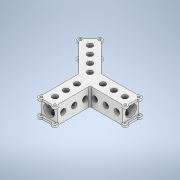
# Autodesk Inventor part: BracketV2
Saved by Autodesk Inventor 2022 (Build 260153000, 153)
## iProperties
Created: 2022-02-05
Part Number: BracketV2
Material: Generic
Document SubType Name: Modeling
Designer: ultra
Density: 1 g/cm^3
Appearance: Smooth - White
Author: ultra
Autodesk Inventor part; units mm, degrees
ref_plane "YZ Plane" through (0, 0, 0) normal (1, 0, 0) x (0, 1, 0)
ref_plane "XZ Plane" through (0, 0, 0) normal (0, 1, 0) x (-1, 0, 0)
ref_plane "XY Plane" through (0, 0, 0) normal (0, 0, 1) x (1, 0, 0)
sketch "Sketch2" plane through (0, 0, 0) normal (1, 0, 0) x (0, 1, 0)
  circle A0 centre (0, 0) radius 12.881
  line L0 (-16, -18.5) -> (16, -18.5)
  line L1 (16, -18.5) -> (16, 18.5)
  line L2 (16, 18.5) -> (-16, 18.5)
  line L3 (-16, 18.5) -> (-16, -18.5)
  line L4 (-16, -18.5) -> (16, 18.5) construction
  line L5 (16, -18.5) -> (-16, 18.5) construction
  dimension "d9" = 25.762
  dimension "d10" = 32
  dimension "d11" = 37
  constraints: 12 end point, 2 midpoint, 2 parallel, 1 centre point, 1 coincident, 1 horizontal, 1 perpendicular
  measures "d9" diameter of A0
  measures "d10" distance of L2.end L1.end
  measures "d11" distance of L1.end L0.end
extrude "Extrusion2" add sketch "Sketch2" along normal blind 76.2
sketch "Sketch3" plane through (0, -16, -18.5) normal (0, 0, -1) x (-1, 0, 0)
  line L0 (0, 0) -> (0, 32) projected
  circle A0 centre (18.5, 16) radius 12.881
  line L1 (0, 32) -> (0, 0)
  line L2 (0, 0) -> (37, 0)
  line L3 (37, 0) -> (37, 32)
  line L4 (37, 32) -> (0, 32)
  line L5 (0, 32) -> (37, 0) construction
  line L6 (0, 0) -> (37, 32) construction
  point P0 (0, 16)
  dimension "d14" = 25.762
  dimension "d15" = 32
  dimension "d16" = 37
  constraints: 12 end point, 2 midpoint, 2 parallel, 1 centre point, 1 coincident, 1 perpendicular
  measures "d14" diameter of A0
  measures "d15" distance of L3.end L2.end
  measures "d16" distance of L2.end L1.end
extrude "Extrusion3" add sketch "Sketch3" against normal blind 113.2
sketch "Sketch4" plane through (76.2, -16, -18.5) normal (0, 0, -1) x (-1, 0, 0)
  circle A0 centre (94.7, 16) radius 12.881 projected
  point P0 (76.2, 16)
extrude "Extrusion4" add sketch "Sketch4" against normal blind 37
sketch "Sketch5" plane through (76.2, 16, 18.5) normal (0, 1, 0) x (1, 0, 0)
  line L0 (-113.2, 37) -> (0, 37) projected
  line L1 (-113.2, 37) -> (-113.2, -76.2) projected
  line L2 (-113.2, 37) -> (-100.1185, 50.0815)
  line L3 (-113.2, 37) -> (-94.7, 37) construction
  line L4 (-113.2, 37) -> (-126.2815, 23.9185)
  line L5 (-113.2, 37) -> (-94.7, 37) construction
  line L6 (-100.1185, 50.0815) -> (-154.0001, 103.963)
  line L7 (-126.2815, 23.9185) -> (-180.163, 77.8001)
  line L8 (-126.2815, 23.9185) -> (-50.0815, 23.9185) construction
  line L9 (-154.0001, 103.963) -> (-180.163, 77.8001)
  line L10 (-100.1185, 50.0815) -> (-87.037, 37)
  line L11 (-126.2815, 23.9185) -> (-113.2, 10.837)
  point P0 (-76.2, 18.5)
  dimension "d21" = 18.5
  dimension "d22" = 45
  dimension "d23" = 18.5
  dimension "d24" = 135
  dimension "d25" = 76.2
  dimension "d26" = 76.2
  dimension "d27" = 135
  constraints: 20 end point, 3 equal length, 3 horizontal, 2 point on line
  measures "d21" distance of L0.start L2.end
  measures "d22" angle of L3 L2
  measures "d23" distance of L0.start L4.end
  measures "d24" angle of L4 L5
  measures "d25" distance of L2.end L6.end
  measures "d26" distance of L4.end L7.end
  measures "d27" angle of L8 L7
extrude "Extrusion5" add sketch "Sketch5" against normal blind 32
sketch "Sketch7" plane through (-77.8001, -16, -85.463) normal (-0.7071068, 0, -0.7071068) x (-0.7071068, 0, 0.7071068)
  line L0 (36.4256, 0.4968) -> (36.4256, 31.5032)
  line L1 (36.4256, 31.5032) -> (0.5744, 31.5032)
  line L2 (0.5744, 31.5032) -> (0.5744, 0.4968)
  line L3 (0.5744, 0.4968) -> (36.4256, 0.4968)
  circle A0 centre (18.5, 16) radius 12.881
  point P0 (5.4185, 16)
  point P1 (36.4256, 16)
  dimension "d131" = 25.762
  constraints: 8 end point, 1 centre point
  measures "d131" diameter of A0
extrude "Extrusion6" cut sketch "Sketch7" against normal blind 101.6 contours A0
sketch "Sketch8" plane through (76.2, 16, 18.5) normal (0, 1, 0) x (1, 0, 0)
  line L0 (-76.2, 0) -> (0, 0) projected
  line L1 (-87.037, 37) -> (0, 37) projected
  line L2 (-87.037, 37) -> (-154.0001, 103.963) projected
  line L3 (-180.163, 77.8001) -> (-113.2, 10.837) projected
  line L4 (-113.2, 10.837) -> (-113.2, -76.2) projected
  line L5 (-76.2, 0) -> (-76.2, -76.2) projected
  line L6 (0, 37) -> (5, 37)
  line L7 (5, 37) -> (5, 0)
  line L8 (5, 0) -> (0, 0)
  line L9 (0, 0) -> (0, 37)
  line L10 (-113.2, -76.2) -> (-76.2, -76.2)
  line L11 (-76.2, -76.2) -> (-76.2, -81.2)
  line L12 (-76.2, -81.2) -> (-113.2, -81.2)
  line L13 (-113.2, -81.2) -> (-113.2, -76.2)
  line L14 (-180.163, 77.8001) -> (-183.6985, 81.3356)
  line L15 (-183.6985, 81.3356) -> (-157.5356, 107.4985)
  line L16 (-157.5356, 107.4985) -> (-154.0001, 103.963)
  point P0 (-76.2, 18.5)
  dimension "d32" = 5
  dimension "d33" = 5
  dimension "d34" = 5
  dimension "d35" = 90
  constraints: 22 end point, 4 parallel, 3 perpendicular, 2 horizontal
  measures "d32" distance of L7.end L8.end
  measures "d33" distance of L10.end L11.end
  measures "d34" distance of L3.start L14.end
  measures "d35" angle of L14 L15
extrude "Extrusion7" add sketch "Sketch8" along normal blind 4.7752
sketch "Sketch9" plane through (76.2, -16, -18.5) normal (0, -1, 0) x (1, 0, 0)
  line L0 (-87.037, 0) -> (0, 0) projected
  line L1 (-76.2, 37) -> (0, 37) projected
  line L2 (-76.2, 37) -> (-76.2, 113.2) projected
  line L3 (-113.2, 26.163) -> (-113.2, 113.2) projected
  line L4 (-113.2, 26.163) -> (-180.163, -40.8001) projected
  line L5 (-154.0001, -66.963) -> (-87.037, 0) projected
  line L6 (-76.2, 118.2) -> (-76.2, 37) projected
  line L7 (-113.2, 113.2) -> (-76.2, 113.2)
  line L8 (-76.2, 113.2) -> (-76.2, 118.2)
  line L9 (-76.2, 118.2) -> (-113.2, 118.2)
  line L10 (-113.2, 118.2) -> (-113.2, 113.2)
  line L11 (-76.2, 37) -> (5, 37) projected
  line L12 (0, 0) -> (5, 0)
  line L13 (5, 0) -> (5, 37)
  line L14 (5, 37) -> (0, 37)
  line L15 (0, 37) -> (0, 0)
  line L16 (-183.6985, -44.3356) -> (-113.2, 26.163) projected
  line L17 (-180.163, -40.8001) -> (-183.6985, -44.3356)
  line L18 (-183.6985, -44.3356) -> (-157.5356, -70.4985)
  line L19 (-157.5356, -70.4985) -> (-154.0001, -66.963)
  point P0 (-76.2, 18.5)
  constraints: 22 end point, 4 parallel, 4 perpendicular, 2 horizontal, 1 collinear
extrude "Extrusion8" add sketch "Sketch9" along normal blind 4.7752
sketch "Sketch10" plane through (76.2, 20.7752, 18.5) normal (0, 1, 0) x (1, 0, 0)
  circle A0 centre (2.5, 34.121) radius 1.5875
  circle A1 centre (2.5, 2.879) radius 1.5875
  line L0 (0, 37.379) -> (0, 0.379)
  line L1 (0, 0.379) -> (5, 0.379)
  line L2 (5, 37.379) -> (5, 0.379)
  line L3 (0, 37.379) -> (5, 37.379)
  line L4 (5, 0) -> (5, 37) projected
  line L5 (0, 18.5) -> (5, 18.5)
  point P0 (-76.2, 18.5)
  dimension "d143" = 15.621
  dimension "d144" = 2.5
  dimension "d145" = 2.5
  dimension "d146" = 15.621
  dimension "d169" = 3.175
  constraints: 10 end point, 2 centre point, 1 midpoint
  measures "d143" distance from line of L5 A0.centre
  measures "d144" distance from line of L2 A1.centre
  measures "d145" distance from line of L2 A0.centre
  measures "d146" distance from line of L5 A1.centre
  measures "d169" diameter of A0
extrude "Extrusion9" cut sketch "Sketch10" against normal blind 279.4 contours A0 | A1
sketch "Sketch11" plane through (76.2, 20.7752, 18.5) normal (0, 1, 0) x (1, 0, 0)
  circle A0 centre (-79.079, -78.7) radius 1.5875
  circle A1 centre (-110.321, -78.7) radius 1.5875
  line L0 (-76.579, -76.2) -> (-113.579, -76.2)
  line L1 (-113.579, -76.2) -> (-113.579, -81.2)
  line L2 (-76.579, -81.2) -> (-113.579, -81.2)
  line L3 (-76.579, -76.2) -> (-76.579, -81.2)
  circle A2 centre (-157.8036, 103.695) radius 1.5875
  circle A3 centre (-179.895, 81.6036) radius 1.5875
  line L4 (-157.5356, 107.4985) -> (-183.6985, 81.3356) projected
  line L5 (-170.5878, 94.3878) -> (-167.0743, 90.8743)
  line L6 (-113.2, -81.2) -> (-76.2, -81.2) projected
  line L7 (-94.7, -76.2) -> (-94.7, -81.2)
  line L8 (-87.037, 37) -> (-157.5356, 107.4985) projected
  line L9 (-183.6985, 81.3356) -> (-113.2, 10.837) projected
  line L10 (-113.2, 10.837) -> (-113.2, -81.2) projected
  point P0 (-76.2, 18.5)
  dimension "d147" = 2.5
  dimension "d148" = 2.5
  dimension "d149" = 15.621
  dimension "d150" = 15.621
  dimension "d151" = 2.5
  dimension "d152" = 2.5
  dimension "d153" = 15.621
  dimension "d154" = 15.621
  dimension "d170" = 2.879
  dimension "d171" = 2.879
  dimension "d172" = 2.879
  constraints: 12 end point, 4 centre point, 1 midpoint
  measures "d147" distance from line of L4 A2.centre
  measures "d148" distance from line of L4 A3.centre
  measures "d149" distance from line of L5 A2.centre
  measures "d150" distance from line of L5 A3.centre
  measures "d151" distance from line of L2 A0.centre
  measures "d152" distance from line of L6 A1.centre
  measures "d153" distance from line of L7 A1.centre
  measures "d154" distance from line of A0.centre L7
  measures "d170" distance from line of L8 A2.centre
  measures "d171" distance from line of L9 A3.centre
  measures "d172" distance from line of L10 A1.centre
extrude "Extrusion10" cut sketch "Sketch11" against normal blind 279.4 contours A0 | A1 | A2 | A3
fillet "Fillet1" radius 3.175 3 edges at (-10.837, 0, -18.5) (0, 0, 18.5) (-37, 0, 7.663)
sketch "Sketch13" plane through (76.2, 20.7752, 18.5) normal (0, 1, 0) x (1, 0, 0)
  line L0 (-157.5356, 107.4985) -> (-183.6985, 81.3356) projected
  line L1 (-113.2, -81.2) -> (-76.2, -81.2) projected
  line L2 (5, 0) -> (5, 37) projected
  line L3 (5, 37) -> (5, 0) projected
  line L4 (5, 18.5) -> (-120.863, 18.5)
  line L5 (-114.1299, 11.767) -> (-183.6985, 81.3356) projected
  line L6 (-76.2, -81.2) -> (-113.2, -81.2) projected
  line L7 (-94.7, -81.2) -> (-95.2395, 19.0395)
  line L8 (-104.3477, 9.9312) -> (-86.1312, 28.1477) projected
  line L9 (-95.2395, 19.0395) -> (-170.6171, 94.4171)
  line L10 (-183.6985, 81.3356) -> (-157.5356, 107.4985) projected
  circle A0 centre (-14.05, 18.5) radius 6.35
  circle A1 centre (-39.45, 18.5) radius 6.35
  circle A2 centre (-64.85, 18.5) radius 6.35
  circle A3 centre (-90.25, 18.5) radius 6.35
  circle A4 centre (-94.8025, -62.15) radius 6.35
  circle A5 centre (-94.9392, -36.7504) radius 6.35
  circle A6 centre (-95.0759, -11.3507) radius 6.35
  circle A7 centre (-95.2126, 14.0489) radius 6.35
  circle A8 centre (-157.1467, 80.9467) radius 6.35
  circle A9 centre (-139.1862, 62.9862) radius 6.35
  circle A10 centre (-121.2257, 45.0257) radius 6.35
  circle A11 centre (-103.2651, 27.0651) radius 6.35
  point P0 (-76.2, 18.5)
  point P1 (-95.1101, -5.0008)
  point P2 (-95.0418, -17.7006)
  point P3 (-94.9734, -30.4005)
  point P4 (-94.9051, -43.1003)
  dimension "d60" = 12.7
  dimension "d61" = 19.05
  dimension "d64" = 25.4
  dimension "d69" = 12.7
  dimension "d70" = 19.05
  dimension "d73" = 25.4
  dimension "d78" = 12.7
  dimension "d79" = 19.05
  dimension "d82" = 25.4
  constraints: 12 centre point, 6 end point, 4 midpoint, 4 point on line, 2 horizontal, 20 other
  measures "d60" diameter of A0
  measures "d61" distance from line of L2 A0.centre
  measures "d64" distance of A0.centre A1.centre
  measures "d69" diameter of A4
  measures "d70" distance from line of L1 A4.centre
  measures "d73" distance of A4.centre A5.centre
  measures "d78" diameter of A8
  measures "d79" distance from line of L0 A8.centre
  measures "d82" distance of A8.centre A9.centre
extrude "Extrusion12" cut sketch "Sketch13" against normal blind 127 contours A8 L9 | L9 A8 | A9 L9 | L9 A9 | A11 L9 | L9 A11 | A10 L9 | L9 A10 | A0 L4 | L4 A0 | A1 L4 | L4 A1 | A2 L4 | L4 A2 | A4 L7 | L7 A4 | A5 L7 | L7 A5 | A6 L7 | L7 A6
sketch "Sketch14" plane through (81.2, 16, -18.5) normal (0, 0, -1) x (-1, 0, 0)
  line L0 (0, 4.7752) -> (90.7219, 4.7752) projected
  line L1 (0, 0) -> (0, 4.7752) projected
  circle A0 centre (19.05, -16) radius 6.35
  circle A1 centre (44.45, -16) radius 6.35
  circle A2 centre (69.85, -16) radius 6.35
  point P0 (81.2, -16)
  dimension "d89" = 12.7
  dimension "d91" = 19.05
  dimension "d94" = 25.4
  constraints: 3 centre point, 1 horizontal, 4 other
  measures "d89" diameter of A0
  measures "d91" distance from line of A0.centre L1
  measures "d94" distance of A0.centre A1.centre
extrude "Extrusion13" cut sketch "Sketch14" against normal blind 50.8
sketch "Sketch15" plane through (-37, 16, 94.7) normal (-1, 0, 0) x (0, 0, 1)
  line L0 (5, 0) -> (5, 4.7752) projected
  line L1 (-85.7219, 4.7752) -> (5, 4.7752) projected
  circle A0 centre (-14.05, -16) radius 6.35
  circle A1 centre (-39.45, -16) radius 6.35
  circle A2 centre (-64.85, -16) radius 6.35
  point P0 (-94.7, -16)
  dimension "d101" = 12.7
  dimension "d102" = 19.05
  dimension "d105" = 25.4
  constraints: 3 centre point, 1 horizontal, 4 other
  measures "d101" diameter of A0
  measures "d102" distance from line of L0 A0.centre
  measures "d105" distance of A0.centre A1.centre
extrude "Extrusion14" cut sketch "Sketch15" against normal blind 50.8
sketch "Sketch16" plane through (-107.4985, 16, -62.8356) normal (-0.7071068, 0, 0.7071068) x (0.7071068, 0, 0.7071068)
  line L0 (0, 4.7752) -> (98.3849, 4.7752) projected
  line L1 (0, 0) -> (0, 4.7752) projected
  circle A0 centre (19.05, -16) radius 6.35
  circle A1 centre (44.45, -16) radius 6.35
  circle A2 centre (69.85, -16) radius 6.35
  point P0 (120.4444, -16)
  dimension "d112" = 12.7
  dimension "d113" = 19.05
  dimension "d116" = 25.4
  constraints: 3 centre point, 1 horizontal, 4 other
  measures "d112" diameter of A0
  measures "d113" distance from line of L1 A0.centre
  measures "d116" distance of A0.centre A1.centre
extrude "Extrusion15" cut sketch "Sketch16" against normal blind 101.6
sketch "Sketch19" plane through (76.2, 20.7752, 18.5) normal (0, 1, 0) x (1, 0, 0)
  circle A0 centre (-157.8036, 103.695) radius 1.5875 projected
  circle A1 centre (-79.079, -78.7) radius 1.5875 projected
  circle A2 centre (-179.895, 81.6036) radius 1.5875 projected
  circle A3 centre (-110.321, -78.7) radius 1.5875 projected
  circle A4 centre (2.5, 2.879) radius 1.5875 projected
  circle A5 centre (2.5, 34.121) radius 1.5875 projected
  line L0 (-87.967, 37.9299) -> (-157.5356, 107.4985) projected
  line L1 (-157.5356, 107.4985) -> (-183.6985, 81.3356) projected
  line L2 (-183.6985, 81.3356) -> (-114.1299, 11.767) projected
  line L3 (-113.2, 9.5219) -> (-113.2, -81.2) projected
  line L4 (-113.2, -81.2) -> (-76.2, -81.2) projected
  line L5 (-76.2, -81.2) -> (-76.2, -3.175) projected
  line L6 (-73.025, 0) -> (5, 0) projected
  line L7 (5, 0) -> (5, 37) projected
  line L8 (5, 37) -> (-85.7219, 37) projected
  circle A6 centre (2.5, 2.879) radius 6
  circle A7 centre (2.5, 34.121) radius 6
  circle A8 centre (-110.321, -78.7) radius 6
  circle A9 centre (-79.079, -78.7) radius 6
  circle A10 centre (-179.895, 81.6036) radius 6
  circle A11 centre (-157.8036, 103.695) radius 6
  point P0 (-76.2, 18.5)
  point P1 (-76.2, -73.4358)
  point P2 (-84.5334, -81.2)
  point P3 (-113.2, -73.4358)
  point P4 (-104.8666, -81.2)
  point P5 (-177.806, 87.2282)
  point P6 (-178.2085, 75.8455)
  point P7 (-152.0455, 102.0085)
  point P8 (-163.4282, 101.606)
  point P9 (5, 8.3334)
  point P10 (-2.7642, 0)
  point P11 (-2.7642, 37)
  point P12 (5, 28.6666)
  dimension "d132" = 12
  dimension "d133" = 12
  dimension "d134" = 12
  dimension "d135" = 12
  dimension "d136" = 12
  dimension "d137" = 12
  constraints: 6 centre point, 6 coincident
  measures "d132" diameter of A6
  measures "d133" diameter of A7
  measures "d134" diameter of A8
  measures "d135" diameter of A9
  measures "d136" diameter of A10
  measures "d137" diameter of A11
extrude "Extrusion17" add sketch "Sketch19" against normal blind 4.7752 contours L0 L1 A11 | L1 L2 A10 | L3 L4 A8 | L4 L5 A9 | L6 L7 A6 | L7 L8 A7 picked at (-161.5779, 104.0552) picked at (-180.2286, 85.3749) picked at (-107.8901, -81.6026) picked at (-81.4972, -81.6185) picked at (5.3897, 5.3199) picked at (5.3897, 31.6801)
sketch "Sketch20" plane through (76.2, -20.7752, -18.5) normal (0, -1, 0) x (1, 0, 0)
  circle A0 centre (-157.8036, -66.695) radius 1.5875 projected
  circle A1 centre (-179.895, -44.6036) radius 1.5875 projected
  circle A2 centre (2.5, 34.121) radius 1.5875 projected
  circle A3 centre (2.5, 2.879) radius 1.5875 projected
  line L0 (-157.5356, -70.4985) -> (-87.967, -0.9299) projected
  line L1 (-85.7219, 0) -> (5, 0) projected
  line L2 (5, 0) -> (5, 37) projected
  line L3 (5, 37) -> (-73.025, 37) projected
  line L4 (-76.2, 40.175) -> (-76.2, 118.2) projected
  line L5 (-76.2, 118.2) -> (-113.2, 118.2) projected
  line L6 (-113.2, 118.2) -> (-113.2, 27.4781) projected
  line L7 (-114.1299, 25.233) -> (-183.6985, -44.3356) projected
  line L8 (-183.6985, -44.3356) -> (-157.5356, -70.4985) projected
  circle A4 centre (-157.8036, -66.695) radius 6
  circle A5 centre (-179.895, -44.6036) radius 6
  circle A6 centre (-110.321, 115.7) radius 1.5875 projected
  circle A7 centre (-110.321, 115.7) radius 6
  circle A8 centre (-79.079, 115.7) radius 1.5875 projected
  circle A9 centre (-79.079, 115.7) radius 6
  circle A10 centre (2.5, 34.121) radius 6
  circle A11 centre (2.5, 2.879) radius 6
  point P0 (-76.2, 18.5)
  point P1 (5, 8.3334)
  point P2 (-2.7642, 0)
  point P3 (-2.7642, 37)
  point P4 (5, 28.6666)
  point P5 (-84.5334, 118.2)
  point P6 (-76.2, 110.4358)
  point P7 (-104.8666, 118.2)
  point P8 (-113.2, 110.4358)
  point P9 (-163.4282, -64.606)
  point P10 (-152.0455, -65.0085)
  point P11 (-178.2085, -38.8455)
  point P12 (-177.806, -50.2282)
  dimension "d163" = 12
  dimension "d164" = 12
  dimension "d165" = 12
  dimension "d166" = 12
  dimension "d167" = 12
  dimension "d168" = 12
  constraints: 6 centre point, 6 coincident
  measures "d163" diameter of A9
  measures "d164" diameter of A7
  measures "d165" diameter of A5
  measures "d166" diameter of A4
  measures "d167" diameter of A10
  measures "d168" diameter of A11
extrude "Extrusion18" add sketch "Sketch20" against normal blind 4.7752 contours L0 A4 L8 | L1 L2 A11 | L2 L3 A10 | L4 L5 A9 | L5 L6 A7 | L7 L8 A5 picked at (-161.5779, -67.0552) picked at (5.3897, 5.3199) picked at (5.3897, 31.6801) picked at (-81.4972, 118.6185) picked at (-107.8901, 118.6026) picked at (-180.2286, -48.3749)
sketch "Sketch21" plane through (76.2, 20.7752, 18.5) normal (0, 1, 0) x (1, 0, 0)
  circle A0 centre (-79.079, -78.7) radius 1.5875 projected
  circle A1 centre (-110.321, -78.7) radius 1.5875 projected
  circle A2 centre (2.5, 2.879) radius 1.5875 projected
  circle A3 centre (2.5, 34.121) radius 1.5875 projected
  arc A4 (-152.0455, 102.0085) -> (-163.4282, 101.606) centre (-157.8036, 103.695) ccw projected
  arc A5 (-177.806, 87.2282) -> (-178.2085, 75.8455) centre (-179.895, 81.6036) ccw projected
  arc A6 (-113.2, -73.4358) -> (-104.8666, -81.2) centre (-110.321, -78.7) ccw projected
  circle A7 centre (-110.321, -78.7) radius 2.925
  circle A8 centre (-79.079, -78.7) radius 1.5875 projected
  circle A9 centre (-79.079, -78.7) radius 2.925
  circle A10 centre (2.5, 34.121) radius 1.5875 projected
  circle A11 centre (2.5, 34.121) radius 2.925
  circle A12 centre (2.5, 2.879) radius 1.5875 projected
  circle A13 centre (2.5, 2.879) radius 2.925
  circle A14 centre (-157.8036, 103.695) radius 2.925
  circle A15 centre (-179.895, 81.6036) radius 2.925
  point P0 (-76.2, 18.5)
  dimension "d155" = 5.85
  dimension "d156" = 5.85
  dimension "d157" = 5.85
  dimension "d158" = 5.85
  dimension "d159" = 5.85
  dimension "d160" = 5.85
  constraints: 6 centre point, 6 coincident
  measures "d155" diameter of A7
  measures "d156" diameter of A9
  measures "d157" diameter of A11
  measures "d158" diameter of A13
  measures "d159" diameter of A14
  measures "d160" diameter of A15
extrude "Extrusion19" cut sketch "Sketch21" against normal blind 5.08
body "Solid2"
